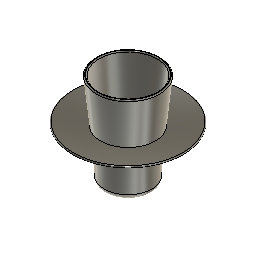
Candle holder for 18mm hole (Autodesk Fusion 360 design; units mm, degrees)
Autodesk Fusion 360 part; units mm, degrees
sketch "Sketch1" plane through (0, 0, 0) normal (0, 0, 1) x (1, 0, 0)
  circle A0 centre (0, 0) radius 9
  dimension "d1" = 18
  constraint coincident A0.centre origin
  measures "d1" diameter of A0
extrude "Extrude1" add sketch "Sketch1" along normal blind 15 makes body 1
sketch "Sketch2" plane through (0, 0, 0) normal (0, 1, 0) x (1, 0, 0)
  circle A0 centre (0, -59.55) radius 45.45
  line L0 (-25, -20) -> (30, -20) construction
  line L1 (0, -10) -> (0, -230)
  circle A1 centre (0, -143.997) radius 126.003
  constraint horizontal L0
  constraint perpendicular L0 L1
revolve "Revolve1" add sketch "Sketch2" angle 360 about axis through (0, 0, 1.75) along (0, 0, 1) separate body contours A0 L1 A1 picked at (4.446, -16.896) makes body 2
fillet "Fillet1" radius 0.3 1 edges at (-20.8787, -8.0981, 20) on bodies 2
ref_plane "WorkPlane1" through (0, 0, 35) normal (0, 0, 1) x (1, 0, 0)
sketch "Sketch3" plane through (0, 0, 15) normal (0, 0, 1) x (-1, 0, 0)
  circle A0 centre (0, 0) radius 9
  circle A1 centre (0, 0) radius 10
  dimension "d9" = 20
  constraint coincident A0.centre A1.centre
  measures "d9" diameter of A1
sketch "Sketch4" plane through (0, 0, 35) normal (0, 0, 1) x (1, 0, 0)
  circle A0 centre (0, 0) radius 12
  circle A1 centre (0, 0) radius 11
  dimension "d10" = 24
  dimension "d11" = 22
  constraint coincident A0.centre A1.centre
  constraint concentric A0 A1
  measures "d10" diameter of A0
  measures "d11" diameter of A1
loft "Loft2" add profiles "Sketch3", "Sketch4" section 1 section 2 separate body makes body 3
loft "Loft3" cut profiles "Sketch3", "Sketch4" section 1 contours A0 section 2 contours A1 bodies 3
fillet "Fillet2" radius 0.4 2 edges at (-11.1879, 4.3394, 35) (-10.2556, 3.9778, 35) on bodies 3
fillet "Fillet3" radius 1 1 edges at (9.3233, 3.6162, 15) on bodies 3
fillet "Fillet4" radius 2 1 edges at (-8.3909, -3.2545, 0) on bodies 1
combine "Combine1" operation add target body 3 tool bodies 2 1
loft "Loft1" [suppressed]
